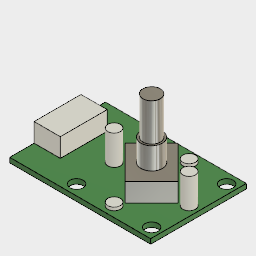
Control_Panel_v4 (Autodesk Fusion 360 archive; units mm, degrees)
design "Encoder"
Autodesk Fusion 360 part; units mm, degrees
note: some values were not read from the file. Chosen so that the rebuilt part matches the saved one: which face or edge a step refers to; how an offset face is resized. Set by a fixed rule: which sketch regions a step uses.
sketch "Sketch1" plane through (0, 0, 0) normal (0, 0, 1) x (1, 0, 0) in component "Encoder"
  line L0 (-22.55, -15.325) -> (22.55, -15.325)
  line L1 (22.55, -15.325) -> (22.55, 15.325)
  line L2 (22.55, 15.325) -> (-22.55, 15.325)
  line L3 (-22.55, 15.325) -> (-22.55, -15.325)
  line L4 (-22.55, 0) -> (22.55, 0) construction
  line L5 (7.55, -15.325) -> (7.55, 15.325) construction
  circle A0 centre (19.55, 12) radius 2.1
  circle A1 centre (7.55, 0) radius 3.425
  circle A2 centre (-4.45, 12) radius 2.1
  circle A3 centre (-4.45, -12) radius 2.1
  circle A4 centre (19.55, -12) radius 2.1
  circle A5 centre (7.55, 0) radius 2.8
  circle A6 centre (19.55, 0) radius 2
  circle A7 centre (7.55, 12) radius 2
  circle A8 centre (-4.45, 0) radius 2
  circle A9 centre (7.55, -12) radius 2
  line L6 (-22.55, -7.5) -> (-14.15, -7.5)
  line L7 (-14.15, -7.5) -> (-14.15, 7.5)
  line L8 (-14.15, 7.5) -> (-22.55, 7.5)
  line L9 (-22.55, 7.5) -> (-22.55, -7.5)
  line L10 (-1.9959, 1.0607) -> (6.4893, 9.5459)
  line L11 (6.4893, 9.5459) -> (17.0959, -1.0607)
  line L12 (17.0959, -1.0607) -> (8.6107, -9.5459)
  line L13 (8.6107, -9.5459) -> (-1.9959, 1.0607)
  line L14 (2.2467, 5.3033) -> (12.8533, -5.3033) construction
  line L15 (19.55, 0) -> (19.55, 12) construction
  dimension "d1" = 30.65
  dimension "d2" = 45.1
  dimension "d3" = 15
  dimension "d4" = 4.2
  dimension "d8" = 360
  dimension "d9" = 6.85
  dimension "d10" = 5.6
  dimension "d11" = 4
  dimension "d14" = 360
  dimension "d15" = 15
  dimension "d16" = 8.4
  dimension "d17" = 15
  dimension "d18" = 12
  dimension "d19" = 45
  dimension "d42" = 12
  dimension "d43" = 12
  measures "d1" distance of L0.start L2.end
  measures "d2" distance of L1.end L2.end
  measures "d3" distance of L1 L5
  measures "d4" diameter of A0
  measures "d9" diameter of A1
  measures "d10" diameter of A5
  measures "d11" diameter of A6
  measures "d15" distance of L6.start L8.end
  measures "d16" distance of L6.start L6.end
  measures "d17" distance of L10.end L11.end
  measures "d18" distance of L10.start L10.end
  measures "d19" angle of L4 L11
  measures "d42" distance of L5.end A0.centre
  measures "d43" distance of L4.end A0.centre
extrude "Extrude1" add sketch "Sketch1" along normal blind 1.56 contours L0 L1 L2 L3 L6 L7 L8 | L3 L6 L7 L8 L9 | A1 | A5 | A6 | A7 | A8 | A9 | L10 L11 L12 L13 makes body 1 in component "Encoder"
extrude "Extrude2" add sketch "Sketch1" along normal blind 6 from surface at 1.56 separate body contours L3 L6 L7 L8 L9 makes body 2 in component "Encoder"
extrude "Extrude3" add sketch "Sketch1" along normal blind 6 from surface at 1.56 separate body contours A1 | A5 | L10 L11 L12 L13 makes body 3 in component "Encoder"
extrude "Extrude4" add sketch "Sketch1" along normal blind 7 from surface at 7.56 contours A1 | A5 bodies 3 in component "Encoder"
extrude "Extrude5" add sketch "Sketch1" along normal blind 12 from surface at 14.56 contours A5 bodies 3 in component "Encoder"
extrude "Extrude6" add sketch "Sketch1" along normal blind 9.5 from surface at 1.56 separate body contours A6 | A8 makes body 4 at (21.5401, -0.1991, 7.8933) makes body 5 at (-2.4599, -0.1991, 7.8933) in component "Encoder"
extrude "Extrude7" add sketch "Sketch1" along normal blind 1 from surface at 1.56 separate body contours A7 | A9 makes body 6 at (9.5401, -12.1991, 2.2267) makes body 7 at (9.5401, 11.8009, 2.2267) in component "Encoder"
component "Encoder" placed x (1, 0, 0) y (0, 1, 0) z (0, 0, 1) at (0, 0, 0)
named bodies: "PCB", "Connector", "Encoder", "LED 1", "LED 2", "LED 3", "LED 4"

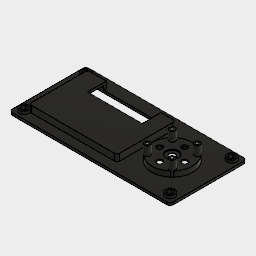
design "Control Panel Back Frame"
Autodesk Fusion 360 part; units mm, degrees
sketch "Sketch1" plane through (0, 0, 0) normal (0, 0, 1) x (1, 0, 0) in component "Control Panel Back Frame"
  line L0 (-64.4, 25.65) -> (15.1, 25.65)
  line L1 (15.1, 25.65) -> (15.1, -25.65)
  circle A0 centre (70.1, -29.65) radius 1.6
  circle A1 centre (70.1, 29.65) radius 1.6
  circle A2 centre (42.5, 0) radius 17.5
  circle A3 centre (-70.1, -29.65) radius 1.6
  line L2 (77.4, -33.95) -> (77.4, 33.95)
  circle A4 centre (-70.1, 29.65) radius 1.6
  line L3 (-74.4, -36.95) -> (74.4, -36.95)
  line L4 (74.4, 36.95) -> (-74.4, 36.95)
  line L5 (-77.4, 0) -> (77.4, 0) construction
  line L6 (-64.4, -25.65) -> (-64.4, 25.65)
  line L7 (0, -36.95) -> (0, 36.95) construction
  line L8 (15.1, -25.65) -> (-64.4, -25.65)
  line L9 (-77.4, 33.95) -> (-77.4, -33.95)
  arc A5 (-74.4, 36.95) -> (-77.4, 33.95) centre (-74.4, 33.95) ccw
  arc A6 (-77.4, -33.95) -> (-74.4, -36.95) centre (-74.4, -33.95) ccw
  arc A7 (74.4, -36.95) -> (77.4, -33.95) centre (74.4, -33.95) ccw
  arc A8 (77.4, 33.95) -> (74.4, 36.95) centre (74.4, 33.95) ccw
  circle A9 centre (42.5, 0) radius 2.8
  circle A10 centre (30.5, 0) radius 2.7
  circle A11 centre (42.5, 0) radius 6.035
  circle A12 centre (30.5, 12) radius 2.825
  line L10 (30.5, 0) -> (30.5, 14.825) construction
  circle A13 centre (42.5, 0) radius 19.61
  circle A14 centre (30.5, -12) radius 2.825
  circle A15 centre (42.5, -12) radius 2.7
  circle A16 centre (54.5, -12) radius 2.825
  circle A17 centre (54.5, 0) radius 2.7
  circle A18 centre (54.5, 12) radius 2.825
  circle A19 centre (42.5, 12) radius 2.7
  circle A20 centre (-70.1, -29.65) radius 4.5
  line L11 (-66.9246, -29.65) -> (-68.5123, -26.9)
  line L12 (-68.5123, -26.9) -> (-71.6877, -26.9)
  line L13 (-71.6877, -26.9) -> (-73.2754, -29.65)
  line L14 (-73.2754, -29.65) -> (-71.6877, -32.4)
  line L15 (-71.6877, -32.4) -> (-68.5123, -32.4)
  line L16 (-68.5123, -32.4) -> (-66.9246, -29.65)
  circle A21 centre (-70.1, 29.65) radius 4.5
  line L17 (-71.6877, 26.9) -> (-73.2754, 29.65)
  line L18 (-73.2754, 29.65) -> (-71.6877, 32.4)
  line L19 (-71.6877, 32.4) -> (-68.5123, 32.4)
  line L20 (-68.5123, 32.4) -> (-66.9246, 29.65)
  line L21 (-68.5123, 26.9) -> (-71.6877, 26.9)
  line L22 (-66.9246, 29.65) -> (-68.5123, 26.9)
  circle A22 centre (70.1, 29.65) radius 4.5
  line L23 (71.6877, 26.9) -> (73.2754, 29.65)
  line L24 (73.2754, 29.65) -> (71.6877, 32.4)
  line L25 (71.6877, 32.4) -> (68.5123, 32.4)
  line L26 (68.5123, 32.4) -> (66.9246, 29.65)
  line L27 (68.5123, 26.9) -> (71.6877, 26.9)
  line L28 (66.9246, 29.65) -> (68.5123, 26.9)
  line L29 (71.6877, -26.9) -> (73.2754, -29.65)
  line L30 (73.2754, -29.65) -> (71.6877, -32.4)
  line L31 (71.6877, -32.4) -> (68.5123, -32.4)
  line L32 (68.5123, -32.4) -> (66.9246, -29.65)
  line L33 (68.5123, -26.9) -> (71.6877, -26.9)
  line L34 (66.9246, -29.65) -> (68.5123, -26.9)
  circle A23 centre (70.1, -29.65) radius 4.5
  circle A24 centre (-70.5, -19.85) radius 3.9
  line L35 (-64.4, -28.15) -> (15.1, -28.15)
  line L36 (17.6, -25.65) -> (17.6, 25.65)
  line L37 (15.1, 28.15) -> (-64.4, 28.15)
  line L38 (-66.9, 25.65) -> (-66.9, -25.65)
  arc A25 (-64.4, 28.15) -> (-66.9, 25.65) centre (-64.4, 25.65) ccw
  arc A26 (-66.9, -25.65) -> (-64.4, -28.15) centre (-64.4, -25.65) ccw
  arc A27 (15.1, -28.15) -> (17.6, -25.65) centre (15.1, -25.65) ccw
  arc A28 (17.6, 25.65) -> (15.1, 28.15) centre (15.1, 25.65) ccw
  circle A29 centre (-70.5, 20.15) radius 3.9
  circle A30 centre (70.5, -19.85) radius 3.9
  circle A31 centre (70.5, 20.15) radius 3.9
  circle A32 centre (30.5, 12) radius 1.5
  circle A33 centre (30.5, -12) radius 1.5
  circle A34 centre (54.5, -12) radius 1.5
  circle A35 centre (54.5, 12) radius 1.5
  line L39 (-48.9, 10.05) -> (3.6, 10.05)
  line L40 (-48.9, 10.05) -> (-48.9, 28.15)
  line L41 (3.6, 10.05) -> (3.6, 28.15)
  point P0 (77.4, -36.95)
  point P1 (-77.4, 36.95)
  point P2 (-64.4, 0)
  point P3 (-77.4, -36.95)
  point P4 (60, 0)
  point P5 (-70.1, -29.65)
  point P6 (22.89, 0)
  dimension "d1" = 73.9
  dimension "d2" = 154.8
  dimension "d3" = 35
  dimension "d4" = 17.4
  dimension "d10" = 13
  dimension "d11" = 11.3
  dimension "d12" = 79.5
  dimension "d14" = 3.2
  dimension "d15" = 7.3
  dimension "d16" = 7.3
  dimension "d19" = 3
  dimension "d20" = 5.6
  dimension "d24" = 5.4
  dimension "d25" = 12.07
  dimension "d27" = 5.65
  dimension "d31" = 39.22
  dimension "d33" = 360
  dimension "d37" = 9
  dimension "d38" = 5.5
  dimension "d39" = 7.8
  dimension "d40" = 6.9
  dimension "d41" = 17.1
  dimension "d42" = 8.8
  dimension "d43" = 10.5
  dimension "d44" = 8.8
  dimension "d47" = 2.5
  dimension "d48" = 2.5
  dimension "d49" = 7.8
  dimension "d50" = 6.9
  dimension "d51" = 16.8
  dimension "d56" = 3
  dimension "d58" = 360
  dimension "d79" = 12
  dimension "d80" = 12
  dimension "d81" = 52.5
  dimension "d82" = 15.5
  dimension "d83" = 15.6
  measures "d1" distance of P1 P3
  measures "d2" distance of P0 P3
  measures "d3" diameter of A2
  measures "d4" distance of P4 L2
  measures "d10" distance of L6 L9
  measures "d11" distance of L0 L4
  measures "d12" distance of L0.start L0.end
  measures "d14" diameter of A3
  measures "d15" distance of P5 L9
  measures "d16" distance of P5 L3
  measures "d19" radius of A5
  measures "d20" diameter of A9
  measures "d24" diameter of A10
  measures "d25" diameter of A11
  measures "d27" diameter of A12
  measures "d31" diameter of A13
  measures "d37" diameter of A20
  measures "d38" distance of L11 L14
  measures "d39" diameter of A24
  measures "d40" distance of L9 A24.centre
  measures "d41" distance of L3 A24.centre
  measures "d42" distance of L3 L35
  measures "d43" distance of L9 L38
  measures "d44" distance of L4 L37
  measures "d47" distance of L1 L36
  measures "d48" radius of A25
  measures "d49" diameter of A29
  measures "d50" distance of L9 A29.centre
  measures "d51" distance of L4 A29.centre
  measures "d56" diameter of A32
  measures "d79" distance of A2.centre L10
  measures "d80" distance of P6 A12.centre
  measures "d81" distance of L39.start L39.end
  measures "d82" distance of L6 L39.start
  measures "d83" distance of L0 L39.start
extrude "Extrude1" add sketch "Sketch1" along normal blind 2.55 contours L0 L1 L6 L8 A20 A21 A24 L35 L36 L37 L38 A25 A26 A27 A28 A29 L40 L41 | L0 L1 L6 L8 L39 L40 L41 | L0 L37 L40 L41 | L0 L39 L40 L41 | A21 A25 | A21 A25 | L38 A29 | L38 A29 | A20 A26 | A20 A26 | A24 L38 | A24 L38 | L2 L3 L4 L9 A5 A6 A7 A8 | L11 L12 L13 L14 L15 L16 | L17 L18 L19 L20 L21 L22 | A22 | L23 L24 L25 L26 L27 L28 | L29 L30 L31 L32 L33 L34 | A23 | A30 | A31 in component "Control Panel Back Frame"
extrude "Extrude8" add sketch "Sketch1" along normal blind 9 contours L0 L1 L6 L8 A20 A21 A24 L35 L36 L37 L38 A25 A26 A27 A28 A29 L40 L41 | L0 L1 L6 L8 L39 L40 L41 | L38 A29 | A24 L38 picked at (-66.8448, 19.8118) picked at (-66.8448, -20.1882) in component "Control Panel Back Frame"
extrude "Extrude9" cut sketch "Sketch1" along normal blind 6.45 contours L0 L1 L6 L8 L39 L40 L41 | L0 L39 L40 L41 in component "Control Panel Back Frame"
extrude "Extrude2" cut sketch "Sketch1" along normal blind 1.3 contours L38 A29 | L38 A29 | A24 L38 | A24 L38 | A30 | A31 in component "Control Panel Back Frame"
extrude "Extrude3" add sketch "Sketch1" along normal blind 16.8 contours A2 A18 A35 | A2 A13 A18 A35 | A2 A13 A16 A34 | A2 A16 A34 | A2 A35 | A2 A35 | A2 A34 | A2 A34 | A2 A12 A32 | A2 A12 A13 A32 | A13 A18 | A13 A16 | A2 A13 A14 A33 | A2 A14 A33 | A2 A32 | A2 A32 | A12 A13 | A2 A33 | A2 A33 | A13 A14 in component "Control Panel Back Frame"
extrude "Extrude4" cut sketch "Sketch1" against normal blind 8 from surface at 16.8 contours A2 A35 | A2 A35 | A2 A34 | A2 A34 | A2 A32 | A2 A32 | A2 A33 | A2 A33 in component "Control Panel Back Frame"
extrude "Extrude5" add sketch "Sketch1" along normal blind 7.8 contours A2 A12 A14 A16 A18 | A2 A13 A16 A18 | A2 A12 A13 A18 | A2 A13 A14 A16 | A2 A12 A13 A14 | A11 in component "Control Panel Back Frame"
extrude "Extrude6" cut sketch "Sketch1" along normal blind 6.3 contours A2 A12 A14 A16 A18 | A2 A18 A35 | A2 A16 A34 | A2 A35 | A2 A34 | A2 A12 A32 | A2 A14 A33 | A2 A32 | A2 A33 | A11 picked at (54.393, 11.893) picked at (54.393, -11.893) picked at (30.6216, 11.9082) picked at (30.6216, -11.9082) in component "Control Panel Back Frame"
extrude "Extrude7" cut sketch "Sketch1" against normal blind 1 from surface at 7.8 contours A11 in component "Control Panel Back Frame"
extrude "Extrude10" add sketch "Sketch1" along normal blind 5 contours A21 A25 | A20 A26 | A22 | A23 picked at (-70.101, 26.3167) picked at (-70.101, -26.3167) in component "Control Panel Back Frame"
extrude "Extrude11" cut sketch "Sketch1" against normal blind 3.45 from surface at 5 contours L11 L12 L13 L14 L15 L16 | L17 L18 L19 L20 L21 L22 | L23 L24 L25 L26 L27 L28 | L29 L30 L31 L32 L33 L34 in component "Control Panel Back Frame"
thread "Thread1" "ISO Metric profile 3.0 M3x0.5 6H" major diameter 3.086 minor diameter 2.529 pitch 0.5 angle 60 resizes the face on face at (31.9981, 11.9252, 11.4667) in component "Control Panel Back Frame"
thread "Thread2" "ISO Metric profile 3.0 M3x0.5 6H" major diameter 3.086 minor diameter 2.529 pitch 0.5 angle 60 resizes the face on face at (54.0223, 13.4219, 11.4667) in component "Control Panel Back Frame"
thread "Thread3" "ISO Metric profile 3.0 M3x0.5 6H" major diameter 3.086 minor diameter 2.529 pitch 0.5 angle 60 resizes the face on face at (53.6862, -10.74, 14.1333) in component "Control Panel Back Frame"
thread "Thread4" "ISO Metric profile 3.0 M3x0.5 6H" major diameter 3.086 minor diameter 2.529 pitch 0.5 angle 60 resizes the face on face at (31.9925, -11.8506, 14.1333) in component "Control Panel Back Frame"
component "Control Panel Back Frame" placed x (1, 0, 0) y (0, 1, 0) z (0, 0, 1) at (0, 0, 0)
equation "d40 = 3 mm + d39 / 2"
equation "d41 = 13.2 mm + d39 / 2"
equation "d49 = d39"
equation "d50 = d40"
equation "d51 = 12.9 mm + d49 / 2"

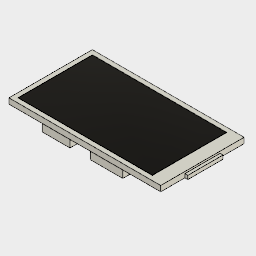
design "LCD and UI Ctrl"
Autodesk Fusion 360 part; units mm, degrees
sketch "Sketch1" plane through (0, 0, 0) normal (0, 0, 1) x (1, 0, 0) in component "LCD and UI Ctrl"
  line L0 (-41, -22.55) -> (41, -22.55)
  line L1 (41, -22.55) -> (41, 22.55)
  line L2 (41, 22.55) -> (-41, 22.55)
  line L3 (-41, 22.55) -> (-41, -22.55)
  line L4 (-41, 0) -> (41, 0) construction
  line L5 (34.05, -20.1) -> (-38.55, -20.1)
  line L6 (-38.55, -20.1) -> (-38.55, 20.1)
  line L7 (-38.55, 20.1) -> (34.05, 20.1)
  line L8 (34.05, 20.1) -> (34.05, -20.1)
  line L9 (-25, -20.55) -> (-10, -20.55)
  line L10 (-10, -20.55) -> (-10, -12.35)
  line L11 (-10, -12.35) -> (-25, -12.35)
  line L12 (-25, -12.35) -> (-25, -20.55)
  line L13 (1, -20.55) -> (18.5, -20.55)
  line L14 (18.5, -20.55) -> (18.5, -12.35)
  line L15 (18.5, -12.35) -> (1, -12.35)
  line L16 (1, -12.35) -> (1, -20.55)
  line L17 (42.6, 9.5) -> (42.6, -9.5)
  line L18 (41, 0) -> (42.6, 0) construction
  line L19 (42.6, 9.5) -> (41, 9.5)
  line L20 (42.6, -9.5) -> (41, -9.5)
  point P0 (-38.55, 0)
  dimension "d1" = 45.1
  dimension "d2" = 82
  dimension "d3" = 72.6
  dimension "d4" = 40.2
  dimension "d5" = 2.45
  dimension "d7" = 2.45
  dimension "d8" = 15
  dimension "d9" = 17.5
  dimension "d10" = 2
  dimension "d11" = 8.2
  dimension "d12" = 16
  dimension "d13" = 11
  dimension "d18" = 1.6
  measures "d1" distance of L0.start L2.end
  measures "d2" distance of L1.end L2.end
  measures "d3" distance of L6.end L7.end
  measures "d4" distance of L6.end L5.end
  measures "d5" distance of L3 L6
  measures "d7" distance of L2 L7
  measures "d8" distance of L9.start L9.end
  measures "d9" distance of L13.start L13.end
  measures "d10" distance of L0 L9
  measures "d11" distance of L9.start L11.end
  measures "d12" distance of L3 L12
  measures "d13" distance of L10 L16
  measures "d18" distance of L4.end L18.end
extrude "Extrude1" add sketch "Sketch1" along normal blind 3 contours L0 L1 L2 L3 | L5 L13 L14 L16 | L5 L9 L10 L12 makes body 1 in component "LCD and UI Ctrl"
extrude "Extrude2" add sketch "Sketch1" against normal blind 6 contours L5 L13 L14 L16 | L5 L14 L15 L16 | L5 L9 L10 L12 | L5 L10 L11 L12 bodies 1 in component "LCD and UI Ctrl"
extrude "Extrude3" add sketch "Sketch1" along normal blind 2 contours L1 L17 L19 L20 bodies 1 in component "LCD and UI Ctrl"
extrude "Extrude4" add sketch "Sketch1" along normal blind 3 separate body contours L5 L6 L7 L8 L10 L11 L12 L14 L15 L16 | L5 L14 L15 L16 | L5 L10 L11 L12 makes body 2 in component "LCD and UI Ctrl"
component "LCD and UI Ctrl" placed x (1, 0, 0) y (0, 1, 0) z (0, 0, 1) at (0, 0, 0)
named bodies: "Screen Space"

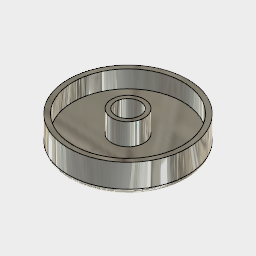
design "Knob"
Autodesk Fusion 360 part; units mm, degrees
sketch "Sketch1" plane through (0, 0, 0) normal (0, 0, 1) x (1, 0, 0) in component "Knob"
  circle A0 centre (0, 0) radius 14.85
  circle A1 centre (0, 0) radius 13.65
  circle A2 centre (0, 0) radius 3.05
  circle A3 centre (0, 0) radius 4.05
  circle A4 centre (0, 0) radius 9.75
  dimension "d1" = 29.7
  dimension "d2" = 1.2
  dimension "d3" = 6.1
  dimension "d4" = 1
  dimension "d15" = 19.5
  measures "d1" diameter of A0
  measures "d3" diameter of A2
  measures "d15" diameter of A4
extrude "Extrude1" add sketch "Sketch1" along normal blind 7.3 contours A0 | A1 | A4 in component "Knob"
extrude "Extrude2" add sketch "Sketch1" along normal blind 8.4 contours A2 | A3 in component "Knob"
extrude "Extrude3" cut sketch "Sketch1" against normal blind 5.8 from surface at 8.4 contours A2 in component "Knob"
extrude "Extrude4" cut sketch "Sketch1" against normal blind 5.4 from surface at 8.4 contours A1 | A4 in component "Knob"
extrude "Extrude5" cut sketch "Sketch1" along normal blind 1.3 contours A2 | A3 | A4 in component "Knob"
fillet "Fillet1" radius 1.5 1 edges at (-13.8451, -5.37, 0) in component "Knob"
chamfer "Chamfer1" distance 3 distance2 1.3 1 edges at (-9.0902, -3.5258, 0) measured on face at (12.064, -1.1476, 0) in component "Knob"
component "Knob" placed x (1, 0, 0) y (0, 1, 0) z (0, 0, 1) at (0, 0, 0)

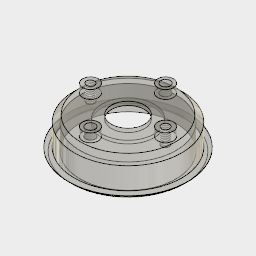
design "Knob Light Pipe"
Autodesk Fusion 360 part; units mm, degrees
sketch "Sketch1" plane through (0, 0, 0) normal (0, 0, 1) x (1, 0, 0) in component "Knob Light Pipe"
  circle A0 centre (0, 0) radius 17
  circle A1 centre (0, 0) radius 15.25
  circle A2 centre (0, 0) radius 18.9
  circle A3 centre (0, 0) radius 5.25
  circle A4 centre (0, 0) radius 8.25
  circle A5 centre (11.9, 0) radius 2.5
  circle A6 centre (11.9, 0) radius 1.5
  line L0 (18.9, 0) -> (-18.9, 0) construction
  circle A7 centre (0, 11.9) radius 1.5
  circle A8 centre (0, 11.9) radius 2.5
  circle A9 centre (-11.9, 0) radius 1.5
  circle A10 centre (-11.9, 0) radius 2.5
  circle A11 centre (0, -11.9) radius 1.5
  circle A12 centre (0, -11.9) radius 2.5
  dimension "d1" = 34
  dimension "d2" = 30.5
  dimension "d3" = 37.8
  dimension "d4" = 10.5
  dimension "d5" = 16.5
  dimension "d6" = 5
  dimension "d7" = 3
  dimension "d8" = 11.9
  dimension "d10" = 360
  measures "d1" diameter of A0
  measures "d2" diameter of A1
  measures "d3" diameter of A2
  measures "d4" diameter of A3
  measures "d5" diameter of A4
  measures "d6" diameter of A5
  measures "d7" diameter of A6
  measures "d8" distance of A0.centre A5.centre
extrude "Extrude1" add sketch "Sketch1" along normal blind 1.1 contours A2 in component "Knob Light Pipe"
extrude "Extrude2" add sketch "Sketch1" along normal blind 10 contours A0 | A1 | A4 | A5 | A7 | A8 | A10 | A11 | A12 in component "Knob Light Pipe"
extrude "Extrude3" cut sketch "Sketch1" along normal blind 7.8 contours A1 | A4 | A5 | A6 | A7 | A8 | A9 | A10 | A11 | A12 in component "Knob Light Pipe"
extrude "Extrude4" add sketch "Sketch1" along normal blind 2.7 from surface at 10 contours A5 | A8 | A10 | A12 in component "Knob Light Pipe"
extrude "Extrude5" cut sketch "Sketch1" along normal blind 1 from surface at 7.8 contours A4 in component "Knob Light Pipe"
thread "Thread1" "ISO Metric profile 3.0 M3x0.5 6H" major diameter 3.086 minor diameter 2.529 pitch 0.5 angle 60 resizes the face on face at (-10.4075, 0.1494, 9.4333) in component "Knob Light Pipe"
thread "Thread2" "ISO Metric profile 3.0 M3x0.5 6H" major diameter 3.086 minor diameter 2.529 pitch 0.5 angle 60 resizes the face on face at (13.3981, 0.0748, 9.4333) in component "Knob Light Pipe"
chamfer "Chamfer1" distance 2 angle 45 1 edges at (-15.8496, -6.1475, 10) in component "Knob Light Pipe"
chamfer "Chamfer2" distance 1 angle 45 1 edges at (-17.621, -6.8345, 0) in component "Knob Light Pipe"
component "Knob Light Pipe" placed x (1, 0, 0) y (0, 1, 0) z (0, 0, 1) at (0, 0, 0)
equation "d8 = ( 28.8 / 2 ) * 1 mm - 2.5 mm"

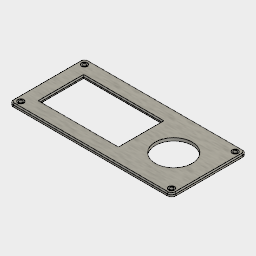
design "Control Panel Cover"
Autodesk Fusion 360 part; units mm, degrees
sketch "Sketch1" plane through (0, 0, 0) normal (0, 0, 1) x (1, 0, 0) in component "Control Panel Cover"
  line L0 (-71.6, -35.1) -> (71.6, -35.1)
  line L1 (75.6, -31.1) -> (75.6, 31.1)
  line L2 (71.6, 35.1) -> (-71.6, 35.1)
  line L3 (-75.6, 31.1) -> (-75.6, -31.1)
  line L4 (-75.6, 0) -> (75.6, 0) construction
  circle A0 centre (42.55, 0) radius 17.15
  line L5 (-64.1, 22.9) -> (18.4, 22.9)
  line L6 (18.4, -22.9) -> (-64.1, -22.9)
  line L7 (-64.1, -22.9) -> (-64.1, 22.9)
  line L8 (20.95, 16) -> (20.95, -16)
  line L9 (20.95, 16) -> (20.4, 16)
  line L10 (20.95, -16) -> (20.4, -16)
  line L11 (18.4, -18) -> (18.4, -22.9)
  line L12 (18.4, 22.9) -> (18.4, 18)
  arc A1 (18.4, 18) -> (20.4, 16) centre (20.4, 18) ccw
  arc A2 (20.4, -16) -> (18.4, -18) centre (20.4, -18) ccw
  line L13 (-61.4, 20.1) -> (11.2, 20.1)
  line L14 (11.2, 20.1) -> (11.2, -20.1)
  line L15 (11.2, -20.1) -> (-61.4, -20.1)
  line L16 (-61.4, -20.1) -> (-61.4, 20.1)
  line L17 (0, -35.1) -> (0, 35.1) construction
  circle A3 centre (-70.1, -29.6) radius 1.6
  circle A4 centre (-70.1, 29.6) radius 1.6
  circle A5 centre (70.1, 29.6) radius 1.6
  circle A6 centre (70.1, -29.6) radius 1.6
  circle A7 centre (-70.1, -29.6) radius 2.7
  circle A8 centre (-70.1, 29.6) radius 2.7
  circle A9 centre (70.1, 29.6) radius 2.7
  circle A10 centre (70.1, -29.6) radius 2.7
  arc A11 (-71.6, 35.1) -> (-75.6, 31.1) centre (-71.6, 31.1) ccw
  arc A12 (-75.6, -31.1) -> (-71.6, -35.1) centre (-71.6, -31.1) ccw
  arc A13 (71.6, -35.1) -> (75.6, -31.1) centre (71.6, -31.1) ccw
  arc A14 (75.6, 31.1) -> (71.6, 35.1) centre (71.6, 31.1) ccw
  point P0 (-75.6, -35.1)
  point P1 (75.6, -35.1)
  point P2 (-75.6, 35.1)
  point P3 (59.7, 0)
  point P4 (-64.1, 0)
  point P5 (20.95, 0)
  point P6 (-61.4, 0)
  dimension "d1" = 70.2
  dimension "d2" = 151.2
  dimension "d3" = 34.3
  dimension "d4" = 15.9
  dimension "d5" = 11.5
  dimension "d6" = 12.2
  dimension "d7" = 82.5
  dimension "d8" = 32
  dimension "d10" = 2
  dimension "d11" = 14.2
  dimension "d12" = 15
  dimension "d13" = 72.6
  dimension "d14" = 85.05
  dimension "d15" = 3.2
  dimension "d16" = 5.5
  dimension "d17" = 5.5
  dimension "d18" = 5.4
  dimension "d27" = 4
  measures "d1" distance of P0 P2
  measures "d2" distance of P0 P1
  measures "d3" diameter of A0
  measures "d4" distance of L1 P3
  measures "d5" distance of L3 P4
  measures "d6" distance of L2 L5
  measures "d7" distance of L5.start L5.end
  measures "d8" distance of L8.start L8.end
  measures "d10" radius of A1
  measures "d11" distance of L3 L16
  measures "d12" distance of L2 L13
  measures "d13" distance of L13.start L13.end
  measures "d14" distance of L7 L8
  measures "d15" diameter of A3
  measures "d16" distance of L3 A3.centre
  measures "d17" distance of L0 A3.centre
  measures "d18" diameter of A7
  measures "d27" radius of A11
extrude "Extrude1" add sketch "Sketch1" along normal blind 2.75 contours L0 L1 L2 L3 A11 A12 A13 A14 | L5 L6 L7 L8 L9 L10 L11 L12 A1 A2 | A7 | A8 | A9 | A10 in component "Control Panel Cover"
extrude "Extrude2" cut sketch "Sketch1" along normal blind 0.5 contours L5 L6 L7 L8 L9 L10 L11 L12 A1 A2 in component "Control Panel Cover"
chamfer "Chamfer1" distance 1 angle 45 8 edges at (74.4284, 33.9284, 2.75) (0, 35.1, 2.75) (-74.4284, 33.9284, 2.75) (-75.6, 0, 2.75) (-74.4284, -33.9284, 2.75) (0, -35.1, 2.75) (74.4284, -33.9284, 2.75) (75.6, 0, 2.75) in component "Control Panel Cover"
chamfer "Chamfer2" distance 1 angle 45 4 edges at (-25.1, 20.1, 2.75) (-61.4, 0, 2.75) (11.2, 0, 2.75) (-25.1, -20.1, 2.75) in component "Control Panel Cover"
extrude "Extrude3" cut sketch "Sketch1" against normal blind 0.25 from surface at 2.75 contours A7 | A8 | A9 | A10 in component "Control Panel Cover"
component "Control Panel Cover" placed x (1, 0, 0) y (0, 1, 0) z (0, 0, 1) at (0, 0, 0)
